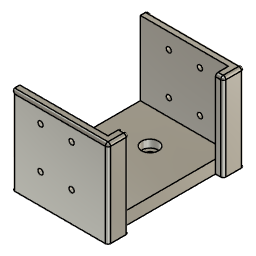
motor_mount v3 (Autodesk Fusion 360 design; units mm, degrees)
Autodesk Fusion 360 part; units mm, degrees
sketch "Sketch1" plane through (0, 0, 0) normal (0, 0, 1) x (1, 0, 0)
  line L0 (0, 0) -> (34, 0)
  line L1 (34, 0) -> (34, 46.5)
  line L2 (34, 46.5) -> (0, 46.5)
  line L3 (0, 46.5) -> (0, 0)
  dimension "d1" = 34
  dimension "d2" = 46.5
  constraint horizontal L0
  constraint vertical L1
  constraint horizontal L2
  constraint vertical L3
  constraint coincident L0.start L3.end
  measures "d1" distance of L0.start L0.end
  measures "d2" distance of L0.start L2.end
extrude "Extrude1" add sketch "Sketch1" along normal blind 5
sketch "Sketch3" plane through (0, 0, 5) normal (0, 0, 1) x (-1, 0, 0)
  line L0 (-34, 0) -> (-34, -46.5)
  line L1 (-17, 0) -> (-17, -46.5)
  circle A0 centre (-17, -13.25) radius 1.6
  circle A1 centre (-17, -33.25) radius 1.6
  line L2 (0, -46.5) -> (0, 0)
  line L3 (0, 0) -> (-34, 0)
  line L4 (-34, -46.5) -> (0, -46.5)
  dimension "d11" = 3.2
  dimension "d12" = 3.2
  dimension "d13" = 20
  constraint coincident L1 A0.centre
  constraint coincident L1 A1.centre
  measures "d11" diameter of A0
  measures "d12" diameter of A1
  measures "d13" distance of A0.centre A1.centre
hole "Hole1" at (17, 13.25, 5) at (17, 33.25, 5) direction (0, 0, -1) diameter 3.2 depth 5 tip angle 180 counterbore diameter 6.5 counterbore depth 3
sketch "Sketch4" plane through (0, 0, 0) normal (0, 0, -1) x (1, 0, 0)
  circle A0 centre (17, -13.25) radius 1.6
  circle A1 centre (17, -33.25) radius 1.6
  line L0 (0, 0) -> (0, -46.5)
  line L1 (0, -46.5) -> (34, -46.5)
  line L2 (34, -46.5) -> (34, 0)
  line L3 (34, 0) -> (0, 0)
  line L4 (0, -46.5) -> (37, -46.5)
  line L5 (37, -46.5) -> (37, -49.5)
  line L6 (37, -49.5) -> (0, -49.5)
  line L7 (0, -49.5) -> (0, -46.5)
  line L8 (0, 0) -> (37, 0)
  line L9 (37, 0) -> (37, 3)
  line L10 (37, 3) -> (0, 3)
  line L11 (0, 3) -> (0, 0)
  line L12 (37, 0) -> (34, 0)
  line L13 (34, 0) -> (34, -5)
  line L14 (34, -5) -> (37, -5)
  line L15 (37, -5) -> (37, 0)
  line L16 (37, -46.5) -> (34, -46.5)
  line L17 (34, -46.5) -> (34, -41.5)
  line L18 (34, -41.5) -> (37, -41.5)
  line L19 (37, -41.5) -> (37, -46.5)
  dimension "d24" = 37
  dimension "d25" = 3
  dimension "d26" = 37
  dimension "d27" = 3
  dimension "d28" = 5
  dimension "d29" = 5
  constraint horizontal L4
  constraint vertical L5
  constraint horizontal L6
  constraint vertical L7
  constraint coincident L0.end L1.start
  constraint horizontal L8
  constraint vertical L9
  constraint horizontal L10
  constraint vertical L11
  constraint coincident L0.start L3.end
  constraint horizontal L12
  constraint vertical L13
  constraint horizontal L14
  constraint vertical L15
  constraint coincident L2 L13.end
  constraint horizontal L16
  constraint vertical L17
  constraint horizontal L18
  constraint vertical L19
  measures "d24" distance of L0.end L4.end
  measures "d25" distance of L0.end L6.end
  measures "d26" distance of L0.start L8.end
  measures "d27" distance of L0.start L10.end
  measures "d28" distance of L4.end L18.end
  measures "d29" distance of L12 L14
extrude "Extrude3" add sketch "Sketch4" against normal blind 33.5 contours L3 L8 L9 L10 L11 L12 | L1 L4 L5 L6 L7 L16 | L2 L8 L12 L13 L14 L15 | L2 L4 L16 L17 L18 L19
sketch "Sketch5" plane through (0, -3, 0) normal (0, -1, 0) x (1, 0, 0)
  line L0 (0, 0) -> (37, 0)
  line L1 (37, 0) -> (37, 33.5)
  line L2 (37, 33.5) -> (0, 33.5)
  line L3 (0, 33.5) -> (0, 0)
  circle A0 centre (11, 27.5) radius 1
  circle A1 centre (23, 27.5) radius 1
  circle A2 centre (11, 11.5) radius 1
  circle A3 centre (23, 11.5) radius 1
  dimension "d32" = 2
  dimension "d33" = 6
  dimension "d34" = 11
  dimension "d37" = 12
  dimension "d38" = -16
  measures "d32" diameter of A0
  measures "d33" distance of L2 A0.centre
  measures "d34" distance of L3 A0.centre
extrude "Extrude4" cut sketch "Sketch5" against normal blind 52.5 contours A0 | A1 | A2 | A3
fillet "Fillet3" radius 1 12 edges at (35.5, 5, 33.5) (37, 1, 33.5) (18.5, -3, 33.5) (37, -3, 16.75) (37, 5, 16.75) (0, -3, 16.75) (37, 41.5, 16.75) (37, 45.5, 33.5) (35.5, 41.5, 33.5) (37, 49.5, 16.75) (18.5, 49.5, 33.5) (0, 49.5, 16.75)
